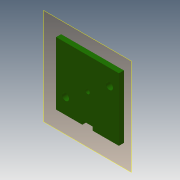
# Autodesk Inventor part: HbSensorBoard02
Saved by Autodesk Inventor 2015 SP1 (Build 190203100, 203)
## iProperties
Created: 2015-05-21
Part Number: HbSensorBoard02
Material: CFRP
Document SubType Name: Modeling
Designer: Yamaura
Density: 1.43 g/cm^3
Appearance: 濃い緑
Author: Yamaura
Autodesk Inventor part; units mm, degrees
ref_plane "YZ Plane" through (0, 0, 0) normal (1, 0, 0) x (0, 1, 0)
ref_plane "XZ Plane" through (0, 0, 0) normal (0, 1, 0) x (-1, 0, 0)
ref_plane "XY Plane" through (0, 0, 0) normal (0, 0, 1) x (1, 0, 0)
ref_plane "作業平面1" through (0, 0, 0) normal (0, 0, 1) x (1, 0, 0)
sketch "スケッチ1" plane through (0, 0, 0) normal (0, 0, 1) x (1, 0, 0)
  line L0 (-12.7, 11.83) -> (-12.7, 13.57) projected
  line L1 (12.3, -13.97) -> (10.56, -13.97) projected
  line L2 (12.7, -11.83) -> (12.7, -13.57) projected
  line L3 (-10, 10) -> (10, 10)
  line L4 (10, 10) -> (10, -10)
  line L5 (10, -10) -> (-10, -10)
  line L6 (-10, -10) -> (-10, 10)
  point P0 (0, 0)
  dimension "d35" = 10
  dimension "d36" = 20
  dimension "d37" = 10
  dimension "d39" = 20
  constraints: 8 end point, 2 parallel, 1 horizontal, 1 perpendicular
  measures "d35" distance from line of L4 point (0, 0)
  measures "d36" distance of L4.end L5.end
  measures "d37" distance from line of L5 point (0, 0)
  measures "d39" distance of L3.end L4.end
extrude "押し出し1" add sketch "スケッチ1" against normal blind 1.6
sketch "スケッチ2" plane through (0, 0, 0) normal (0, 0, 1) x (1, 0, 0)
  circle A0 centre (-7, -5) radius 1.1
  circle A1 centre (7, 5) radius 1.1
  point P0 (0, 0)
  dimension "d2" = 2.2
  dimension "d3" = 2.2
  dimension "d4" = 7
  dimension "d7" = 7
  dimension "d43" = 5
  dimension "d44" = 5
  constraints: 2 centre point
  measures "d2" diameter of A0
  measures "d3" diameter of A1
  measures "d4" horizontal distance of point (0, 0) A0.centre
  measures "d7" horizontal distance of A1.centre point (0, 0)
  measures "d43" vertical distance of point (0, 0) A1.centre
  measures "d44" vertical distance of A0.centre point (0, 0)
extrude "押し出し2" cut sketch "スケッチ2" along normal mid plane 20
sketch "スケッチ5" plane through (0, 0, 0) normal (0, 0, 1) x (1, 0, 0)
  circle A0 centre (0, 0) radius 0.7
  line L0 (1.65, -8.85) -> (-1.65, -8.85)
  line L1 (-1.65, -8.85) -> (-1.65, -14.7)
  line L2 (-1.65, -14.7) -> (1.65, -14.7)
  line L3 (1.65, -14.7) -> (1.65, -8.85)
  dimension "d16" = 1.4
  dimension "d40" = 1.65
  dimension "d41" = 3.3
  dimension "d42" = 8.85
  constraints: 8 end point, 2 parallel, 1 centre point, 1 coincident, 1 horizontal, 1 perpendicular
  measures "d16" diameter of A0
  measures "d40" distance from line of L3 point (0, 0)
  measures "d41" distance of L1.end L2.end
  measures "d42" distance from line of L0 point (0, 0)
extrude "押し出し5" cut sketch "スケッチ5" against normal blind 20
